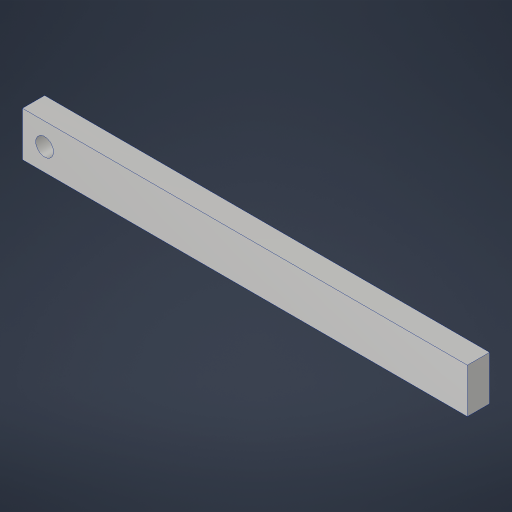
# Autodesk Inventor part: CL6-007
Saved by Autodesk Inventor 2023.4 (Build 274418000, 418)
## iProperties
Created: 2025-03-15
Part Number: CL6-007
Material: Aluminum 6061
Document SubType Name: Modeling
Designer: brand
Density: 2.7 g/cm^3
Appearance: Aluminum - Flat
Author: brand
Autodesk Inventor part; units mm, degrees
ref_plane "YZ Plane" through (0, 0, 0) normal (1, 0, 0) x (0, 1, 0)
ref_plane "XZ Plane" through (0, 0, 0) normal (0, 1, 0) x (-1, 0, 0)
ref_plane "XY Plane" through (0, 0, 0) normal (0, 0, 1) x (1, 0, 0)
sketch "Sketch1" plane through (0, 0, 0) normal (0, 0, 1) x (1, 0, 0)
  line L0 (-63.5, -6.35) -> (63.5, -6.35)
  line L1 (63.5, -6.35) -> (63.5, 6.35)
  line L2 (63.5, 6.35) -> (-63.5, 6.35)
  line L3 (-63.5, 6.35) -> (-63.5, -6.35)
  line L4 (-63.5, -6.35) -> (63.5, 6.35) construction
  line L5 (63.5, -6.35) -> (-63.5, 6.35) construction
  point P0 (0, 0)
  point P1 (-57.15, 0)
  dimension "d0" = 127
  dimension "d1" = 12.7
  dimension "d2" = 6.35
  constraints: 12 end point, 2 midpoint, 2 parallel, 1 horizontal, 1 horizontal alignment, 1 perpendicular
  measures "d0" distance of L2.end L1.end
  measures "d1" distance of L1.end L0.end
  measures "d2" distance from line of point (-57.15, 0) L3
extrude "Extrusion1" add sketch "Sketch1" against normal blind 6.35
hole "Hole1" at (-57.15, 0, 0) direction (0, 0, -1) diameter 5.1054 end through all clearance for "Flat Head Machine Screw (82)" size "#10" standard "Ansi Unified Screw Threads"
body "Solid1"
